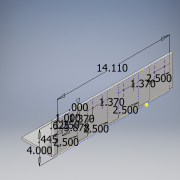
# Autodesk Inventor part: ubracket
Saved by Autodesk Inventor 2017 (Build 210142000, 142)
## iProperties
Created: 2018-03-08
Part Number: ubracket
Material: Generic
Document SubType Name: Sheet Metal
Designer: Zara
Density: 1 g/cm^3
Sheet Metal Rule: Default
Appearance: Default
Author: Zara
Autodesk Inventor part; units mm, degrees
ref_plane "YZ Plane" through (0, 0, 0) normal (1, 0, 0) x (0, 1, 0)
ref_plane "XZ Plane" through (0, 0, 0) normal (0, 1, 0) x (-1, 0, 0)
ref_plane "XY Plane" through (0, 0, 0) normal (0, 0, 1) x (1, 0, 0)
sketch "Sketch1" plane through (0, 0, 0) normal (0, 1, 0) x (-1, 0, 0)
  line L0 (59.2667, 296.3333) -> (-42.3333, 296.3333)
  line L1 (-42.3333, 296.3333) -> (-42.3333, -84.6667)
  line L2 (-42.3333, -84.6667) -> (59.2667, -84.6667)
  line L3 (59.2667, -84.6667) -> (59.2667, 296.3333)
  point P0 (0, 0)
  dimension "d0" = 101.6
  dimension "d1" = 381
  measures "d0" distance of L1.end L2.end
  measures "d1" distance of L0.end L1.end
extrude "Plate1" add sketch "Sketch1" along normal blind 6.35
sketch "Sketch2" plane through (35.9833, 0, -84.6667) normal (1, 0, 0) x (0, 1, 0)
  line L0 (0, 381) -> (0, 0)
  line L1 (0, 0) -> (101.6, 0)
  line L2 (101.6, 0) -> (101.6, 381)
  line L3 (101.6, 381) -> (0, 381)
  constraints: 6 end point, 1 horizontal, 1 perpendicular, 1 vertical
edge flange "Flange1" height 101.6 angle 90 thickness 6.35 bend radius 0.0254 thickness toward (1, 0, 0) relief tear relief width 6.35 relief depth 3.175 edges at (42.3333, 6.35, 105.8333) wall of the first edge with corners at (35.9833, 0, 296.3333) (35.9833, 0, -84.6667) (35.9833, 101.6, -84.6667) (35.9833, 101.6, 296.3333)
bend "Bend1"
corner "Corner1"
sketch "Sketch3" plane through (42.3333, 101.6, 296.3333) normal (1, 0, 0) x (0, 0, -1)
  line L0 (11.303, 0) -> (369.697, 0) construction
  line L1 (369.697, 0) -> (369.697, -101.6) construction
  line L2 (369.697, -101.6) -> (11.303, -101.6) construction
  line L3 (11.303, -101.6) -> (11.303, 0) construction
  line L4 (0, -95.2246) -> (0, 0) construction
  line L5 (0, 0) -> (381, 0) construction
  line L6 (11.303, 0) -> (74.803, 0) construction
  line L7 (74.803, 0) -> (74.803, -95.25) construction
  line L8 (74.803, -95.25) -> (11.303, -95.25) construction
  line L9 (11.303, -95.25) -> (11.303, 0) construction
  line L10 (109.601, 0) -> (173.101, 0) construction
  line L11 (173.101, 0) -> (173.101, -95.25) construction
  line L12 (173.101, -95.25) -> (109.601, -95.25) construction
  line L13 (109.601, -95.25) -> (109.601, 0) construction
  line L14 (207.899, 0) -> (271.399, 0) construction
  line L15 (271.399, 0) -> (271.399, -95.25) construction
  line L16 (271.399, -95.25) -> (207.899, -95.25) construction
  line L17 (207.899, -95.25) -> (207.899, 0) construction
  line L18 (306.197, 0) -> (369.697, 0) construction
  line L19 (369.697, 0) -> (369.697, -95.25) construction
  line L20 (369.697, -95.25) -> (306.197, -95.25) construction
  line L21 (306.197, -95.25) -> (306.197, 0) construction
  line L22 (27.178, -25.4) -> (58.928, -25.4) construction
  line L23 (125.6792, -25.4) -> (157.4292, -25.4) construction
  line L24 (224.1804, -25.4) -> (255.9304, -25.4) construction
  line L25 (322.6816, -25.4) -> (354.4316, -25.4) construction
  point P0 (296.3333, -101.6)
  dimension "d13" = 358.394
  dimension "d14" = 11.303
  dimension "d15" = 101.6
  dimension "d16" = 0
  dimension "d17" = 63.5
  dimension "d18" = 63.5
  dimension "d19" = 34.798
  dimension "d20" = 63.5
  dimension "d21" = 34.798
  dimension "d22" = 63.5
  dimension "d23" = 34.798
  dimension "d24" = 25.4
  dimension "d25" = 31.75
  dimension "d26" = 15.875
  dimension "d36" = 98.5012
  constraints: 48 end point, 10 parallel, 7 horizontal, 5 perpendicular, 3 point on line, 1 collinear, 8 other
  measures "d13" distance of L0.start L0.end
  measures "d14" distance between parallel lines of L4 L3
  measures "d15" distance of L2.end L0.start
  measures "d16" distance between parallel lines of L5 L0
  measures "d17" distance of L7.end L8.end
  measures "d18" distance of L11.end L12.end
  measures "d19" distance between parallel lines of L7 L13
  measures "d20" distance of L15.end L16.end
  measures "d21" distance between parallel lines of L11 L17
  measures "d22" distance between parallel lines of L19 L21
  measures "d23" distance between parallel lines of L15 L21
  measures "d24" distance between parallel lines of L6 L22
  measures "d25" distance of L22.start L22.end
  measures "d26" distance from line of L9 L22.start
  measures "d36" distance of L22.start L23.start
hole "Hole1" at (42.3333, 76.2, 269.1553) at (42.3333, 76.2, 237.4053) at (42.3333, 76.2, 138.9041) at (42.3333, 76.2, 170.6541) at (42.3333, 76.2, 72.1529) at (42.3333, 76.2, 40.4029) at (42.3333, 76.2, -26.3483) at (42.3333, 76.2, -58.0983) direction (-1, 0, 0) diameter 3.9624 depth 13.6144 tip angle 118 thread size "10-32 UNF" class "2B" standard "ANSI Unified Screw Threads"
sketch "Sketch4" plane through (0, 6.35, 0) normal (0, 1, 0) x (1, 0, 0)
  line L0 (-59.2667, -296.3333) -> (-59.2667, 84.6667) projected
  line L1 (-59.2667, 84.6667) -> (35.9579, 84.6667) projected
  point P0 (-11.6417, 59.2667)
  point P1 (-11.6417, -6.7733)
  point P2 (-11.6417, -72.8133)
  point P3 (-11.6417, -138.8533)
  point P4 (-11.6417, -204.8933)
  point P5 (-11.6417, -270.9333)
  dimension "d41" = 47.625
  dimension "d42" = 25.4
  dimension "d45" = 66.04
  constraints: 1 vertical, 5 other
  measures "d41" distance from line of point (-11.642, 59.267) L0
  measures "d42" distance from line of point (-11.642, 59.267) L1
  measures "d45" distance of point (-11.642, 59.267) point (-11.642, -6.773)
hole "Hole2" at (-11.6417, 6.35, -59.2667) at (-11.6417, 6.35, 6.7733) at (-11.6417, 6.35, 72.8133) at (-11.6417, 6.35, 138.8533) at (-11.6417, 6.35, 204.8933) at (-11.6417, 6.35, 270.9333) direction (0, -1, 0) diameter 3.9624 depth 13.6144 tip angle 118 thread size "10-32 UNF" class "2B" standard "ANSI Unified Screw Threads"
equation "\"d3\" = BendReliefWidth"
equation "\"d4\" = BendReliefDepth"
equation "\"d5\" = MinimumRemnant"
equation "\"d6\" = BendRadius"
equation "\"d10\" = CornerReliefSize"
equation "\"d11\" = GapSize"
equation "\"d12\" = JacobiRadiusSize"
equation "\"BendRadius\" = Thickness"
equation "\"BendReliefWidth\" = Thickness"
equation "\"BendReliefDepth\" = 0.5 * Thickness"
equation "\"CornerReliefSize\" = 4 * Thickness"
equation "\"MinimumRemnant\" = 2 * Thickness"
equation "\"TransitionRadius\" = BendRadius"
equation "\"JacobiRadiusSize\" = Thickness"
equation "\"GapSize\" = Thickness"
equation "\"d2\" = BendRadius"
equation "\"Thickness\" = 6.35"
body "Solid1"
